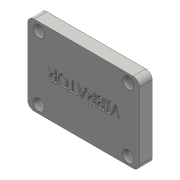
# Autodesk Inventor part: MPU6050_CASE_TOP
Saved by Autodesk Inventor 2016 (Build 200138000, 138)
## iProperties
Created: 2015-05-21
Part Number: MPU6050_CASE_TOP
Material: Generic
Document SubType Name: Modeling
Designer: Admin
Density: 1 g/cm^3
Appearance: Default
Author: Admin
Autodesk Inventor part; units mm, degrees
ref_plane "YZ Plane" through (0, 0, 0) normal (1, 0, 0) x (0, 1, 0)
ref_plane "XZ Plane" through (0, 0, 0) normal (0, 1, 0) x (-1, 0, 0)
ref_plane "XY Plane" through (0, 0, 0) normal (0, 0, 1) x (1, 0, 0)
sketch "Skizze1" plane through (0, 0, 0) normal (0, 1, 0) x (-1, 0, 0)
  line L0 (0, 0) -> (-35, 0)
  line L1 (-35, 0) -> (-35, -25)
  line L2 (-35, -25) -> (0, -25)
  line L3 (0, -25) -> (0, 0)
  dimension "d0" = 35
  dimension "d1" = 25
  constraints: 8 end point, 2 parallel, 1 horizontal, 1 perpendicular
  measures "d0" distance of L2.end L1.end
  measures "d1" distance of L1.end L0.end
extrude "Extrusion1" add sketch "Skizze1" along normal blind 4
fillet "Rundung1" radius 2 1 edges at (35, 2, 0)
fillet "Rundung2" radius 2 1 edges at (0, 2, 0)
fillet "Rundung3" radius 2 1 edges at (0, 2, -25)
fillet "Rundung4" radius 2 1 edges at (35, 2, -25)
sketch "Skizze11" plane through (0, 4, 0) normal (0, 1, 0) x (1, 0, 0)
  circle A0 centre (3.5, 2.5) radius 1.75
  circle A1 centre (3.5, 22.5) radius 1.75
  circle A2 centre (31.5, 2.5) radius 1.75
  circle A3 centre (31.5, 22.5) radius 1.75
  point P0 (0, 0)
  dimension "d36" = 3.5
  dimension "d37" = 3.5
  dimension "d38" = 3.5
  dimension "d39" = 3.5
  constraints: 4 centre point
  measures "d36" diameter of A0
  measures "d37" diameter of A1
  measures "d38" diameter of A2
  measures "d39" diameter of A3
extrude "Extrusion11" cut sketch "Skizze11" against normal blind 10
sketch "Skizze13" plane through (0, 0, 0) normal (0, -1, 0) x (1, 0, 0)
  line L0 (28.9923, -14.0838) -> (6.4097, -14.0838) construction
  line L1 (6.4097, -14.0838) -> (6.4097, -10.4363) construction
  line L2 (6.4097, -10.4363) -> (28.9923, -10.4363) construction
  line L3 (28.9923, -10.4363) -> (28.9923, -14.0838) construction
  line L4 (26.0993, -14.01) -> (27.3047, -10.51)
  line L5 (27.3047, -10.51) -> (27.8068, -10.51)
  line L6 (27.8068, -10.51) -> (29.0122, -14.01)
  line L7 (29.0122, -14.01) -> (28.513, -14.01)
  line L8 (28.513, -14.01) -> (27.543, -11.1028)
  line L9 (27.543, -11.1028) -> (26.573, -14.01)
  line L10 (26.573, -14.01) -> (26.0993, -14.01)
  line L11 (24.545, -10.51) -> (25.9008, -10.51)
  line L12 (25.9008, -10.51) -> (25.9008, -10.8674)
  line L13 (25.9008, -10.8674) -> (25.4555, -10.8674)
  line L14 (25.4555, -10.8674) -> (25.4555, -13.6526)
  line L15 (25.4555, -13.6526) -> (25.9008, -13.6526)
  line L16 (25.9008, -13.6526) -> (25.9008, -14.01)
  line L17 (25.9008, -14.01) -> (24.545, -14.01)
  line L18 (24.545, -14.01) -> (24.545, -13.6526)
  line L19 (24.545, -13.6526) -> (24.9903, -13.6526)
  line L20 (24.9903, -13.6526) -> (24.9903, -10.8674)
  line L21 (24.9903, -10.8674) -> (24.545, -10.8674)
  line L22 (24.545, -10.8674) -> (24.545, -10.51)
  spline S0 degree 2 poles (21.5953, -11.585) (21.5953, -11.324) (21.7938, -10.9241) (21.9583, -10.7936) knots 0 0 0 1 2 2 2
  spline S1 degree 2 poles (21.9583, -10.7936) (22.1568, -10.6405) (22.6078, -10.51) (22.9652, -10.51) knots 0 0 0 1 2 2 2
  line L23 (22.9652, -10.51) -> (23.9692, -10.51)
  line L24 (23.9692, -10.51) -> (23.9692, -14.01)
  line L25 (23.9692, -14.01) -> (23.0418, -14.01)
  spline S2 degree 2 poles (23.0418, -14.01) (22.6674, -14.01) (22.293, -13.9618) (22.1228, -13.8682) knots 0 0 0 1 2 2 2
  spline S3 degree 2 poles (22.1228, -13.8682) (21.9328, -13.7689) (21.7598, -13.4427) (21.7598, -13.2215) knots 0 0 0 1 2 2 2
  spline S4 degree 2 poles (21.7598, -13.2215) (21.7598, -12.9748) (22.0207, -12.5833) (22.2504, -12.4727) knots 0 0 0 1 2 2 2
  line L26 (22.2504, -12.4727) -> (22.2504, -12.4557)
  spline S5 degree 2 poles (22.2504, -12.4557) (21.9385, -12.3706) (21.5953, -11.9197) (21.5953, -11.585) knots 0 0 0 1 2 2 2
  spline S6 degree 2 poles (22.0803, -11.5651) (22.0803, -11.7637) (22.1937, -12.0189) (22.3639, -12.1097) knots 0 0 0 1 2 2 2
  spline S7 degree 2 poles (22.3639, -12.1097) (22.4745, -12.1664) (22.7355, -12.2004) (22.9765, -12.2004) knots 0 0 0 1 2 2 2
  line L27 (22.9765, -12.2004) -> (23.5041, -12.2004)
  line L28 (23.5041, -12.2004) -> (23.5041, -10.9071)
  line L29 (23.5041, -10.9071) -> (23.1269, -10.9071)
  spline S8 degree 2 poles (23.1269, -10.9071) (22.8205, -10.9071) (22.4688, -10.9638) (22.3327, -11.0546) knots 0 0 0 1 2 2 2
  spline S9 degree 2 poles (22.3327, -11.0546) (22.2022, -11.1482) (22.0803, -11.3808) (22.0803, -11.5651) knots 0 0 0 1 2 2 2
  spline S10 degree 2 poles (22.2448, -13.1563) (22.2448, -13.2811) (22.3299, -13.4683) (22.4235, -13.5222) knots 0 0 0 1 2 2 2
  spline S11 degree 2 poles (22.4235, -13.5222) (22.5369, -13.5846) (22.812, -13.6129) (23.0588, -13.6129) knots 0 0 0 1 2 2 2
  line L30 (23.0588, -13.6129) -> (23.5041, -13.6129)
  line L31 (23.5041, -13.6129) -> (23.5041, -12.589)
  line L32 (23.5041, -12.589) -> (22.9765, -12.589)
  spline S12 degree 2 poles (22.9765, -12.589) (22.7581, -12.589) (22.5511, -12.6344) (22.4405, -12.7053) knots 0 0 0 1 2 2 2
  spline S13 degree 2 poles (22.4405, -12.7053) (22.3327, -12.7734) (22.2448, -12.9918) (22.2448, -13.1563) knots 0 0 0 1 2 2 2
  line L33 (18.4243, -10.51) -> (19.0284, -10.51)
  line L34 (19.0284, -10.51) -> (20.1346, -11.9026)
  line L35 (20.1346, -11.9026) -> (20.6678, -11.9026)
  line L36 (20.6678, -11.9026) -> (20.6678, -10.51)
  line L37 (20.6678, -10.51) -> (21.1329, -10.51)
  line L38 (21.1329, -10.51) -> (21.1329, -14.01)
  line L39 (21.1329, -14.01) -> (20.231, -14.01)
  spline S14 degree 2 poles (20.231, -14.01) (19.9303, -14.01) (19.5248, -13.9448) (19.3404, -13.8257) knots 0 0 0 1 2 2 2
  spline S15 degree 2 poles (19.3404, -13.8257) (19.156, -13.7065) (18.9433, -13.335) (18.9433, -13.0598) knots 0 0 0 1 2 2 2
  spline S16 degree 2 poles (18.9433, -13.0598) (18.9433, -12.6769) (19.3347, -12.1579) (19.6694, -12.0331) knots 0 0 0 1 2 2 2
  line L40 (19.6694, -12.0331) -> (18.4243, -10.51)
  spline S17 degree 2 poles (19.4283, -13.023) (19.4283, -13.1761) (19.5361, -13.4116) (19.6496, -13.4881) knots 0 0 0 1 2 2 2
  spline S18 degree 2 poles (19.6496, -13.4881) (19.7488, -13.5534) (20.0126, -13.6073) (20.2055, -13.6073) knots 0 0 0 1 2 2 2
  line L41 (20.2055, -13.6073) -> (20.6678, -13.6073)
  line L42 (20.6678, -13.6073) -> (20.6678, -12.2912)
  line L43 (20.6678, -12.2912) -> (20.2594, -12.2912)
  spline S19 degree 2 poles (20.2594, -12.2912) (20.058, -12.2912) (19.7375, -12.3621) (19.6269, -12.4727) knots 0 0 0 1 2 2 2
  spline S20 degree 2 poles (19.6269, -12.4727) (19.5248, -12.5692) (19.4283, -12.8415) (19.4283, -13.023) knots 0 0 0 1 2 2 2
  line L44 (18.5235, -10.51) -> (17.3436, -14.01)
  line L45 (17.3436, -14.01) -> (16.7707, -14.01)
  line L46 (16.7707, -14.01) -> (15.5908, -10.51)
  line L47 (15.5908, -10.51) -> (16.0815, -10.51)
  line L48 (16.0815, -10.51) -> (16.3991, -11.4885)
  line L49 (16.3991, -11.4885) -> (17.735, -11.4885)
  line L50 (17.735, -11.4885) -> (18.0527, -10.51)
  line L51 (18.0527, -10.51) -> (18.5235, -10.51)
  line L52 (16.5268, -11.8856) -> (17.0685, -13.5335)
  line L53 (17.0685, -13.5335) -> (17.6074, -11.8856)
  line L54 (17.6074, -11.8856) -> (16.5268, -11.8856)
  line L55 (14.4421, -10.51) -> (14.4421, -13.5959)
  line L56 (14.4421, -13.5959) -> (15.6163, -13.5959)
  line L57 (15.6163, -13.5959) -> (15.6163, -14.01)
  line L58 (15.6163, -14.01) -> (12.8027, -14.01)
  line L59 (12.8027, -14.01) -> (12.8027, -13.5959)
  line L60 (12.8027, -13.5959) -> (13.9769, -13.5959)
  line L61 (13.9769, -13.5959) -> (13.9769, -10.51)
  line L62 (13.9769, -10.51) -> (14.4421, -10.51)
  spline S21 degree 2 poles (9.9721, -13.6101) (9.7735, -13.3775) (9.5523, -12.6968) (9.5523, -12.26) knots 0 0 0 1 2 2 2
  spline S22 degree 2 poles (9.5523, -12.26) (9.5523, -11.8346) (9.7679, -11.1453) (9.9721, -10.9128) knots 0 0 0 1 2 2 2
  spline S23 degree 2 poles (9.9721, -10.9128) (10.1876, -10.6688) (10.7577, -10.4363) (11.1009, -10.4363) knots 0 0 0 1 2 2 2
  spline S24 degree 2 poles (11.1009, -10.4363) (11.4555, -10.4363) (12.0227, -10.6774) (12.2298, -10.9128) knots 0 0 0 1 2 2 2
  spline S25 degree 2 poles (12.2298, -10.9128) (12.4312, -11.1453) (12.6467, -11.8289) (12.6467, -12.26) knots 0 0 0 1 2 2 2
  spline S26 degree 2 poles (12.6467, -12.26) (12.6467, -12.6996) (12.4283, -13.369) (12.2269, -13.6101) knots 0 0 0 1 2 2 2
  spline S27 degree 2 poles (12.2269, -13.6101) (12.0227, -13.8427) (11.4526, -14.0838) (11.1009, -14.0838) knots 0 0 0 1 2 2 2
  spline S28 degree 2 poles (11.1009, -14.0838) (10.7436, -14.0838) (10.1706, -13.8342) (9.9721, -13.6101) knots 0 0 0 1 2 2 2
  spline S29 degree 2 poles (10.0373, -12.26) (10.0373, -12.606) (10.1876, -13.1421) (10.3238, -13.318) knots 0 0 0 1 2 2 2
  spline S30 degree 2 poles (10.3238, -13.318) (10.4628, -13.4995) (10.8542, -13.681) (11.0981, -13.681) knots 0 0 0 1 2 2 2
  spline S31 degree 2 poles (11.0981, -13.681) (11.3505, -13.681) (11.7306, -13.5051) (11.8752, -13.318) knots 0 0 0 1 2 2 2
  spline S32 degree 2 poles (11.8752, -13.318) (12.0142, -13.1393) (12.1617, -12.6004) (12.1617, -12.26) knots 0 0 0 1 2 2 2
  spline S33 degree 2 poles (12.1617, -12.26) (12.1617, -11.5708) (11.5831, -10.839) (11.0981, -10.839) knots 0 0 0 1 2 2 2
  spline S34 degree 2 poles (11.0981, -10.839) (10.6131, -10.839) (10.0373, -11.5708) (10.0373, -12.26) knots 0 0 0 1 2 2 2
  line L63 (6.3331, -10.51) -> (6.9372, -10.51)
  line L64 (6.9372, -10.51) -> (8.0434, -11.9026)
  line L65 (8.0434, -11.9026) -> (8.5766, -11.9026)
  line L66 (8.5766, -11.9026) -> (8.5766, -10.51)
  line L67 (8.5766, -10.51) -> (9.0418, -10.51)
  line L68 (9.0418, -10.51) -> (9.0418, -14.01)
  line L69 (9.0418, -14.01) -> (8.1398, -14.01)
  spline S35 degree 2 poles (8.1398, -14.01) (7.8392, -14.01) (7.4336, -13.9448) (7.2492, -13.8257) knots 0 0 0 1 2 2 2
  spline S36 degree 2 poles (7.2492, -13.8257) (7.0649, -13.7065) (6.8521, -13.335) (6.8521, -13.0598) knots 0 0 0 1 2 2 2
  spline S37 degree 2 poles (6.8521, -13.0598) (6.8521, -12.6769) (7.2436, -12.1579) (7.5782, -12.0331) knots 0 0 0 1 2 2 2
  line L70 (7.5782, -12.0331) -> (6.3331, -10.51)
  spline S38 degree 2 poles (7.3372, -13.023) (7.3372, -13.1761) (7.4449, -13.4116) (7.5584, -13.4881) knots 0 0 0 1 2 2 2
  spline S39 degree 2 poles (7.5584, -13.4881) (7.6577, -13.5534) (7.9214, -13.6073) (8.1143, -13.6073) knots 0 0 0 1 2 2 2
  line L71 (8.1143, -13.6073) -> (8.5766, -13.6073)
  line L72 (8.5766, -13.6073) -> (8.5766, -12.2912)
  line L73 (8.5766, -12.2912) -> (8.1682, -12.2912)
  spline S40 degree 2 poles (8.1682, -12.2912) (7.9668, -12.2912) (7.6463, -12.3621) (7.5357, -12.4727) knots 0 0 0 1 2 2 2
  spline S41 degree 2 poles (7.5357, -12.4727) (7.4336, -12.5692) (7.3372, -12.8415) (7.3372, -13.023) knots 0 0 0 1 2 2 2
  point P0 (0, 0)
  constraints: 2 other
extrude "Extrusion13" cut sketch "Skizze13" against normal blind 1
